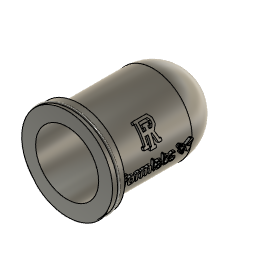
POP_body_derated (Autodesk Fusion 360 design; units mm, degrees)
Autodesk Fusion 360 part; units mm, degrees
sketch "Sketch1" plane through (0, 0, 0) normal (0, 1, 0) x (1, 0, 0)
  circle A0 centre (0, 0) radius 25.65
  circle A1 centre (0, 0) radius 31.75
  dimension "d1" = 51.3
  dimension "d2" = 6.1
  constraint coincident A0.centre A1.centre
  measures "d1" diameter of A0
extrude "Extrude1" add sketch "Sketch1" along normal blind 70 makes body 1
sketch "Sketch2" plane through (0, 0, 0) normal (0, 0, 1) x (1, 0, 0)
  line L0 (0, 0) -> (0, 97.6409) construction
  line L1 (0, 69.4626) -> (31, 69.4626)
  arc A0 (0, 95.1126) -> (-25.65, 69.4626) centre (0, 69.4626) ccw
  arc A1 (0, 101.2126) -> (-31.75, 69.4626) centre (0, 69.4626) ccw
  line L2 (0, 69.4626) -> (-31.75, 69.4626) construction
  line L3 (31, 69.4626) -> (21, 69.4626)
  line L4 (-25.65, 69.4626) -> (-31.75, 69.4626)
  line L5 (0, 95.1126) -> (0, 101.2126)
  dimension "d7" = 31.75
  dimension "d8" = 25.65
  constraint coincident L0.start origin
  constraint vertical L0
  constraint coincident L1.start L0
  constraint coincident L1.start A0.centre
  constraint perpendicular L0 L1
  constraint concentric A0 A1
  constraint coincident L1 L3.end
  constraint perpendicular L0 L2
  constraint coincident L2 A0.end
  measures "d7" radius of A1
  measures "d8" radius of A0
revolve "Revolve1" add sketch "Sketch2" angle 360 about axis through (0, 0, 0) along (0, 1, 0) bodies 1
sketch "Sketch3" plane through (0, 0, 0) normal (0, -1, 0) x (1, 0, 0)
  circle A0 centre (0, 0) radius 25.65
  circle A1 centre (0, 0) radius 31.75
  circle A2 centre (0, 0) radius 25.146 construction
  circle A3 centre (0, 0) radius 28.702 construction
  dimension "d10" = 50.292
  dimension "d11" = 57.404
  constraint coincident A0.centre A1.centre
  measures "d10" diameter of A2
  measures "d11" diameter of A3
ref_plane "WorkPlane1" through (0, 37.2468, -31.75) normal (0, 0, -1) x (1, 0, 0)
sketch "Sketch5" plane through (0, 0, 0) normal (0, -1, 0) x (1, 0, 0)
  circle A0 centre (0, 0) radius 37
  circle A1 centre (0, 0) radius 30.8058
  dimension "d31" = 74
  constraint coincident A0.centre A1.centre
  constraint concentric A0 A1
  measures "d31" diameter of A0
extrude "Extrude3" add sketch "Sketch5" against normal blind 10 bodies 1
coil "CoilPrimitive1" add diameter 74 section circle size 2 on centre turns 1.5 pitch 6.66667 right hand placed x (1, 0, 0) y (0, 0, -1) z (0, 1, 0) at (0, 0, 0) separate body makes body 2
move_body "Move1" bodies 2 to x (1, 0, 0) y (0, 1, 0) z (0, 0, 1) at (0, -1.5, 0)
combine "Combine1" operation add target body 1 tool bodies 2
sketch "Sketch7" plane through (0, 0, 0) normal (0, -1, 0) x (1, 0, 0)
  circle A0 centre (0, 0) radius 25.65
  circle A1 centre (0, 0) radius 50.9902
  spline S0 degree 3 poles (-26.163, -26.163) (-26.1604, -26.1604) (-26.1574, -26.1584) (-26.1496, -26.1548) (-26.1447, -26.1537) (-26.1307, -26.1522) (-26.1207, -26.1533) (-26.0884, -26.1593) (-26.0612, -26.1697) (-25.9436, -26.2231) (-25.8159, -26.3056) (-24.8505, -26.9737) (-23.1166, -28.4335) (-15.2241, -33.4022) (-10.4173, -34.7745) (-2.6703, -36.1642) (1.5215, -36.2078) (5.6316, -35.5568) knots 3.244354 3.244354 3.244354 3.244354 3.253489 3.253489 3.265817 3.265817 3.288767 3.288767 3.348492 3.348492 3.563904 3.563904 4.976735 4.976735 7.989432 7.989432 11.394709 11.394709 11.394709 11.394709
  spline S1 degree 3 poles (5.6316, -35.5568) (6.3802, -35.4382) (7.1261, -35.2966) (12.4413, -34.1173) (16.7708, -32.2508) (24.9958, -26.7102) (27.9306, -23.4279) (30.9522, -19.5432) (31.772, -18.3009) (32.5635, -17.1873) (32.7513, -16.9397) (32.8911, -16.8205) (32.9135, -16.8052) (32.9389, -16.796) (32.9458, -16.7943) (32.9569, -16.7943) (32.9612, -16.795) (32.9659, -16.797) (32.9666, -16.7973) (32.9672, -16.7976) knots 11.394709 11.394709 11.394709 11.394709 12.01493 12.01493 15.836449 15.836449 20.097613 20.097613 22.736598 22.736598 23.856469 23.856469 24.088678 24.088678 24.16644 24.16644 24.216158 24.216158 24.224748 24.224748 24.224748 24.224748
  arc A2 (32.9672, -16.7976) -> (-26.163, -26.163) centre (0, 0) ccw
  constraint concentric A0 A1
extrude "Extrude4" cut sketch "Sketch7" along normal blind 15 contours A1 | S0 S1 A2 bodies 1
ref_plane "WorkPlane3" through (31.75, 49.8809, 0) normal (1, 0, 0) x (0, 0, 1)
sketch "Sketch14" plane through (31.75, 0, 0) normal (1, 0, 0) x (0, 1, 0)
  spline S0 degree 3 poles (15.6914, -0.4908) (15.6818, -0.5681) (15.6432, -0.6164) (15.5562, -0.6164) knots 0 0 0 0 1 1 1 1
  spline S1 degree 3 poles (15.5562, -0.6164) (15.5369, -0.6164) (15.5079, -0.6164) (15.4596, -0.6067) knots 0 0 0 0 1 1 1 1
  spline S2 degree 3 poles (15.4596, -0.6067) (15.3244, -0.5874) (15.0637, -0.5391) (14.8125, -0.5391) knots 0 0 0 0 1 1 1 1
  spline S3 degree 3 poles (14.8125, -0.5391) (14.5614, -0.5391) (14.4069, -0.5681) (14.3006, -0.655) knots 0 0 0 0 1 1 1 1
  spline S4 degree 3 poles (14.3006, -0.655) (14.2041, -0.742) (14.1654, -0.8868) (14.1654, -1.0897) knots 0 0 0 0 1 1 1 1
  line L0 (14.1654, -1.0897) -> (14.1654, -1.6885)
  line L1 (14.1654, -1.6885) -> (15.4983, -1.6885)
  spline S5 degree 3 poles (15.4983, -1.6885) (15.5949, -1.6885) (15.6721, -1.7561) (15.6721, -1.8527) knots 0 0 0 0 1 1 1 1
  line L2 (15.6721, -1.8527) -> (15.6721, -2.8571)
  spline S6 degree 3 poles (15.6721, -2.8571) (15.6721, -2.9537) (15.5949, -3.0117) (15.4983, -3.0117) knots 0 0 0 0 1 1 1 1
  line L3 (15.4983, -3.0117) -> (14.1654, -3.0117)
  line L4 (14.1654, -3.0117) -> (14.1654, -7.213)
  spline S7 degree 3 poles (14.1654, -7.213) (14.1654, -7.3096) (14.0882, -7.3772) (13.9819, -7.3772) knots 0 0 0 0 1 1 1 1
  line L5 (13.9819, -7.3772) -> (12.4366, -7.3772)
  spline S8 degree 3 poles (12.4366, -7.3772) (12.3304, -7.3772) (12.2531, -7.3096) (12.2531, -7.213) knots 0 0 0 0 1 1 1 1
  line L6 (12.2531, -7.213) -> (12.2531, -3.0117)
  line L7 (12.2531, -3.0117) -> (11.4128, -3.0117)
  spline S9 degree 3 poles (11.4128, -3.0117) (11.3066, -3.0117) (11.2293, -2.9537) (11.2293, -2.8571) knots 0 0 0 0 1 1 1 1
  line L8 (11.2293, -2.8571) -> (11.2293, -1.8527)
  spline S10 degree 3 poles (11.2293, -1.8527) (11.2293, -1.7561) (11.3066, -1.6885) (11.4128, -1.6885) knots 0 0 0 0 1 1 1 1
  line L9 (11.4128, -1.6885) -> (12.2531, -1.6885)
  line L10 (12.2531, -1.6885) -> (12.2531, -1.0027)
  spline S11 degree 3 poles (12.2531, -1.0027) (12.2531, 0.1756) (12.8712, 0.7744) (14.1944, 0.7744) knots 0 0 0 0 1 1 1 1
  spline S12 degree 3 poles (14.1944, 0.7744) (15.054, 0.7744) (15.5466, 0.6488) (15.7108, 0.5909) knots 0 0 0 0 1 1 1 1
  spline S13 degree 3 poles (15.7108, 0.5909) (15.817, 0.5619) (15.846, 0.4653) (15.8267, 0.4074) knots 0 0 0 0 1 1 1 1
  line L11 (15.8267, 0.4074) -> (15.6914, -0.4908)
  spline S14 degree 3 poles (18.7725, -7.696) (16.2516, -7.696) (15.9329, -6.4017) (15.9329, -4.7212) knots 0 0 0 0 1 1 1 1
  spline S15 degree 3 poles (15.9329, -4.7212) (15.9329, -3.0406) (16.2516, -1.7368) (18.7725, -1.7368) knots 0 0 0 0 1 1 1 1
  spline S16 degree 3 poles (18.7725, -1.7368) (21.2933, -1.7368) (21.6217, -3.0503) (21.6217, -4.7212) knots 0 0 0 0 1 1 1 1
  spline S17 degree 3 poles (21.6217, -4.7212) (21.6217, -6.4017) (21.2933, -7.696) (18.7725, -7.696) knots 0 0 0 0 1 1 1 1
  spline S18 degree 3 poles (18.7725, -2.9827) (17.9129, -2.9827) (17.8742, -3.4849) (17.8742, -4.7212) knots 0 0 0 0 1 1 1 1
  spline S19 degree 3 poles (17.8742, -4.7212) (17.8742, -5.9575) (17.9225, -6.45) (18.7725, -6.45) knots 0 0 0 0 1 1 1 1
  spline S20 degree 3 poles (18.7725, -6.45) (19.6417, -6.45) (19.6707, -5.9478) (19.6707, -4.7212) knots 0 0 0 0 1 1 1 1
  spline S21 degree 3 poles (19.6707, -4.7212) (19.6707, -3.4753) (19.632, -2.9827) (18.7725, -2.9827) knots 0 0 0 0 1 1 1 1
  spline S22 degree 3 poles (25.6106, -3.0986) (24.9924, -3.0986) (24.4612, -3.1662) (24.3646, -3.1855) knots 0 0 0 0 1 1 1 1
  line L12 (24.3646, -3.1855) -> (24.3646, -7.3772)
  spline S23 degree 3 poles (24.3646, -7.3772) (24.3646, -7.4738) (24.297, -7.5414) (24.1908, -7.5414) knots 0 0 0 0 1 1 1 1
  line L13 (24.1908, -7.5414) -> (22.6358, -7.5414)
  spline S24 degree 3 poles (22.6358, -7.5414) (22.5392, -7.5414) (22.4619, -7.4738) (22.4619, -7.3772) knots 0 0 0 0 1 1 1 1
  line L14 (22.4619, -7.3772) -> (22.4619, -2.5867)
  spline S25 degree 3 poles (22.4619, -2.5867) (22.4619, -2.2004) (22.8096, -2.0748) (23.4567, -1.9396) knots 0 0 0 0 1 1 1 1
  spline S26 degree 3 poles (23.4567, -1.9396) (23.9783, -1.8334) (24.722, -1.7464) (25.3981, -1.7464) knots 0 0 0 0 1 1 1 1
  line L15 (25.3981, -1.7464) -> (25.5816, -1.7464)
  spline S27 degree 3 poles (25.5816, -1.7464) (25.6782, -1.7464) (25.7361, -1.7657) (25.7747, -1.814) knots 0 0 0 0 1 1 1 1
  spline S28 degree 3 poles (25.7747, -1.814) (25.8037, -1.843) (25.8327, -1.901) (25.8327, -1.9879) knots 0 0 0 0 1 1 1 1
  line L16 (25.8327, -1.9879) -> (25.8327, -2.8668)
  spline S29 degree 3 poles (25.8327, -2.8668) (25.8327, -2.9827) (25.8327, -3.0986) (25.6106, -3.0986) knots 0 0 0 0 1 1 1 1
  line L17 (35.1916, -7.5607) -> (33.6366, -7.5607)
  spline S30 degree 3 poles (33.6366, -7.5607) (33.5304, -7.5607) (33.4628, -7.4931) (33.4628, -7.3965) knots 0 0 0 0 1 1 1 1
  line L18 (33.4628, -7.3965) -> (33.4628, -3.7167)
  spline S31 degree 3 poles (33.4628, -3.7167) (33.4628, -3.1469) (33.1634, -2.9634) (32.7384, -2.9634) knots 0 0 0 0 1 1 1 1
  spline S32 degree 3 poles (32.7384, -2.9634) (32.3907, -2.9634) (31.9754, -3.0406) (31.8691, -3.06) knots 0 0 0 0 1 1 1 1
  line L19 (31.8691, -3.06) -> (31.8691, -7.3965)
  spline S33 degree 3 poles (31.8691, -7.3965) (31.8691, -7.4931) (31.7919, -7.5607) (31.6856, -7.5607) knots 0 0 0 0 1 1 1 1
  line L20 (31.6856, -7.5607) -> (30.1306, -7.5607)
  spline S34 degree 3 poles (30.1306, -7.5607) (30.0244, -7.5607) (29.9568, -7.4931) (29.9568, -7.3965) knots 0 0 0 0 1 1 1 1
  line L21 (29.9568, -7.3965) -> (29.9568, -3.7167)
  spline S35 degree 3 poles (29.9568, -3.7167) (29.9568, -3.1469) (29.7057, -2.9634) (29.2807, -2.9634) knots 0 0 0 0 1 1 1 1
  spline S36 degree 3 poles (29.2807, -2.9634) (28.9427, -2.9634) (28.4694, -3.0406) (28.3632, -3.06) knots 0 0 0 0 1 1 1 1
  line L22 (28.3632, -3.06) -> (28.3632, -7.3965)
  spline S37 degree 3 poles (28.3632, -7.3965) (28.3632, -7.4931) (28.2956, -7.5607) (28.1893, -7.5607) knots 0 0 0 0 1 1 1 1
  line L23 (28.1893, -7.5607) -> (26.6343, -7.5607)
  spline S38 degree 3 poles (26.6343, -7.5607) (26.5281, -7.5607) (26.4605, -7.4931) (26.4605, -7.3965) knots 0 0 0 0 1 1 1 1
  line L24 (26.4605, -7.3965) -> (26.4605, -2.6157)
  spline S39 degree 3 poles (26.4605, -2.6157) (26.4605, -2.2197) (26.7985, -2.0941) (27.4649, -1.9589) knots 0 0 0 0 1 1 1 1
  spline S40 degree 3 poles (27.4649, -1.9589) (28.0058, -1.8527) (28.8364, -1.7464) (29.5222, -1.7464) knots 0 0 0 0 1 1 1 1
  spline S41 degree 3 poles (29.5222, -1.7464) (30.2176, -1.7464) (30.6812, -1.9106) (30.9902, -2.1038) knots 0 0 0 0 1 1 1 1
  spline S42 degree 3 poles (30.9902, -2.1038) (31.2027, -2.0265) (32.1299, -1.7464) (33.0668, -1.7464) knots 0 0 0 0 1 1 1 1
  spline S43 degree 3 poles (33.0668, -1.7464) (34.4672, -1.7464) (35.3848, -2.0458) (35.3848, -3.456) knots 0 0 0 0 1 1 1 1
  line L25 (35.3848, -3.456) -> (35.3848, -7.4062)
  spline S44 degree 3 poles (35.3848, -7.4062) (35.3655, -7.4931) (35.2979, -7.5607) (35.1916, -7.5607) knots 0 0 0 0 1 1 1 1
  spline S45 degree 3 poles (38.5431, -7.242) (38.5431, -7.3193) (38.4948, -7.3289) (38.4561, -7.3483) knots 0 0 0 0 1 1 1 1
  spline S46 degree 3 poles (38.4561, -7.3483) (38.3402, -7.4062) (38.0698, -7.4738) (37.6738, -7.4738) knots 0 0 0 0 1 1 1 1
  spline S47 degree 3 poles (37.6738, -7.4738) (37.017, -7.4738) (36.5728, -7.1647) (36.5728, -6.3631) knots 0 0 0 0 1 1 1 1
  line L26 (36.5728, -6.3631) -> (36.5728, 0.4557)
  spline S48 degree 3 poles (36.5728, 0.4557) (36.5728, 0.5426) (36.6307, 0.6005) (36.708, 0.6199) knots 0 0 0 0 1 1 1 1
  line L27 (36.708, 0.6199) -> (37.2971, 0.7744)
  spline S49 degree 3 poles (37.2971, 0.7744) (37.3744, 0.7937) (37.442, 0.7358) (37.442, 0.6488) knots 0 0 0 0 1 1 1 1
  line L28 (37.442, 0.6488) -> (37.442, -6.3341)
  spline S50 degree 3 poles (37.442, -6.3341) (37.442, -6.7205) (37.7124, -6.7784) (37.9346, -6.7784) knots 0 0 0 0 1 1 1 1
  spline S51 degree 3 poles (37.9346, -6.7784) (38.0891, -6.7784) (38.2436, -6.7591) (38.3209, -6.7398) knots 0 0 0 0 1 1 1 1
  line L29 (38.3209, -6.7398) -> (38.3692, -6.7301)
  spline S52 degree 3 poles (38.3692, -6.7301) (38.3982, -6.7301) (38.4465, -6.7398) (38.4561, -6.8074) knots 0 0 0 0 1 1 1 1
  line L30 (38.4561, -6.8074) -> (38.5334, -7.1744)
  spline S53 degree 3 poles (38.5334, -7.1744) (38.5431, -7.2227) (38.5431, -7.2324) (38.5431, -7.242) knots 0 0 0 0 1 1 1 1
  spline S54 degree 3 poles (42.6961, -7.5318) (42.3774, -7.609) (41.8559, -7.696) (41.2667, -7.696) knots 0 0 0 0 1 1 1 1
  spline S55 degree 3 poles (41.2667, -7.696) (40.3202, -7.696) (38.7555, -7.667) (38.7555, -5.9092) knots 0 0 0 0 1 1 1 1
  spline S56 degree 3 poles (38.7555, -5.9092) (38.7555, -4.4797) (39.5379, -4.3832) (40.6486, -4.2093) knots 0 0 0 0 1 1 1 1
  line L31 (40.6486, -4.2093) -> (42.7251, -3.8713)
  line L32 (42.7251, -3.8713) -> (42.7251, -3.3594)
  spline S57 degree 3 poles (42.7251, -3.3594) (42.7251, -3.0117) (42.7155, -2.7316) (42.3291, -2.5867) knots 0 0 0 0 1 1 1 1
  spline S58 degree 3 poles (42.3291, -2.5867) (42.1166, -2.4998) (41.8172, -2.4611) (41.3343, -2.4611) knots 0 0 0 0 1 1 1 1
  spline S59 degree 3 poles (41.3343, -2.4611) (40.494, -2.4611) (39.7697, -2.664) (39.3061, -2.7702) knots 0 0 0 0 1 1 1 1
  spline S60 degree 3 poles (39.3061, -2.7702) (39.1998, -2.7895) (39.1515, -2.7799) (39.1322, -2.693) knots 0 0 0 0 1 1 1 1
  line L33 (39.1322, -2.693) -> (39.0356, -2.21)
  spline S61 degree 3 poles (39.0356, -2.21) (39.0163, -2.1135) (39.1129, -2.0652) (39.1419, -2.0555) knots 0 0 0 0 1 1 1 1
  spline S62 degree 3 poles (39.1419, -2.0555) (39.4896, -1.9299) (40.4361, -1.7175) (41.4309, -1.7175) knots 0 0 0 0 1 1 1 1
  spline S63 degree 3 poles (41.4309, -1.7175) (42.2132, -1.7175) (42.7155, -1.8237) (43.0342, -1.9975) knots 0 0 0 0 1 1 1 1
  spline S64 degree 3 poles (43.0342, -1.9975) (43.5944, -2.2873) (43.604, -2.7992) (43.604, -3.3111) knots 0 0 0 0 1 1 1 1
  line L34 (43.604, -3.3111) -> (43.604, -6.4114)
  spline S65 degree 3 poles (43.604, -6.4114) (43.604, -7.1841) (43.4495, -7.3579) (42.6961, -7.5318) knots 0 0 0 0 1 1 1 1
  line L35 (42.7348, -4.557) -> (40.6003, -4.9144)
  spline S66 degree 3 poles (40.6003, -4.9144) (40.1174, -5.0013) (39.6538, -5.0786) (39.6538, -5.8705) knots 0 0 0 0 1 1 1 1
  spline S67 degree 3 poles (39.6538, -5.8705) (39.6538, -6.9523) (40.552, -7.0295) (41.2764, -7.0295) knots 0 0 0 0 1 1 1 1
  spline S68 degree 3 poles (41.2764, -7.0295) (41.7593, -7.0295) (42.2712, -6.9619) (42.7348, -6.8171) knots 0 0 0 0 1 1 1 1
  line L36 (42.7348, -6.8171) -> (42.7348, -4.557)
  spline S69 degree 3 poles (45.7288, -1.8527) (46.0283, -1.7657) (46.8878, -1.5533) (47.5833, -1.5533) knots 0 0 0 0 1 1 1 1
  spline S70 degree 3 poles (47.5833, -1.5533) (49.399, -1.5533) (49.9109, -2.4708) (49.9109, -4.5184) knots 0 0 0 0 1 1 1 1
  spline S71 degree 3 poles (49.9109, -4.5184) (49.9109, -6.6239) (49.3314, -7.5125) (47.3418, -7.5125) knots 0 0 0 0 1 1 1 1
  spline S72 degree 3 poles (47.3418, -7.5125) (46.5595, -7.5125) (45.8544, -7.3869) (45.4874, -7.2613) knots 0 0 0 0 1 1 1 1
  spline S73 degree 3 poles (45.4874, -7.2613) (44.9369, -7.0778) (44.9176, -6.8074) (44.9176, -6.4114) knots 0 0 0 0 1 1 1 1
  line L37 (44.9176, -6.4114) -> (44.9176, 0.4653)
  spline S74 degree 3 poles (44.9176, 0.4653) (44.9176, 0.5523) (44.9658, 0.5812) (45.0528, 0.6102) knots 0 0 0 0 1 1 1 1
  line L38 (45.0528, 0.6102) -> (45.6419, 0.7647)
  spline S75 degree 3 poles (45.6419, 0.7647) (45.7385, 0.7937) (45.7868, 0.6971) (45.7868, 0.6392) knots 0 0 0 0 1 1 1 1
  line L39 (45.7868, 0.6392) -> (45.7868, -1.2539)
  line L40 (45.7868, -1.2539) -> (45.7288, -1.8527)
  spline S76 degree 3 poles (47.4384, -2.2583) (46.8396, -2.2583) (45.98, -2.4611) (45.7868, -2.5191) knots 0 0 0 0 1 1 1 1
  line L41 (45.7868, -2.5191) -> (45.7868, -6.6432)
  spline S77 degree 3 poles (45.7868, -6.6432) (45.9027, -6.6818) (46.4919, -6.8364) (47.3225, -6.8364) knots 0 0 0 0 1 1 1 1
  spline S78 degree 3 poles (47.3225, -6.8364) (48.5877, -6.8364) (49.0127, -6.2569) (49.0127, -4.5473) knots 0 0 0 0 1 1 1 1
  spline S79 degree 3 poles (49.0127, -4.5473) (49.0127, -2.7992) (48.7036, -2.2583) (47.4384, -2.2583) knots 0 0 0 0 1 1 1 1
  spline S80 degree 3 poles (52.3834, -7.696) (51.4176, -7.696) (50.587, -7.4062) (50.4421, -7.3483) knots 0 0 0 0 1 1 1 1
  spline S81 degree 3 poles (50.4421, -7.3483) (50.3842, -7.3289) (50.3359, -7.2903) (50.3648, -7.1744) knots 0 0 0 0 1 1 1 1
  line L42 (50.3648, -7.1744) -> (50.4614, -6.7591)
  spline S82 degree 3 poles (50.4614, -6.7591) (50.4807, -6.6818) (50.5194, -6.6142) (50.6353, -6.6625) knots 0 0 0 0 1 1 1 1
  spline S83 degree 3 poles (50.6353, -6.6625) (50.6643, -6.6722) (51.4659, -6.9716) (52.4028, -6.9716) knots 0 0 0 0 1 1 1 1
  spline S84 degree 3 poles (52.4028, -6.9716) (53.33, -6.9716) (53.8708, -6.6818) (53.8708, -6.0154) knots 0 0 0 0 1 1 1 1
  spline S85 degree 3 poles (53.8708, -6.0154) (53.8708, -5.1172) (53.1658, -5.1462) (52.3158, -5.0206) knots 0 0 0 0 1 1 1 1
  spline S86 degree 3 poles (52.3158, -5.0206) (51.775, -4.9337) (50.4035, -4.8371) (50.4035, -3.4077) knots 0 0 0 0 1 1 1 1
  spline S87 degree 3 poles (50.4035, -3.4077) (50.4035, -2.0072) (51.6687, -1.7175) (52.6249, -1.7175) knots 0 0 0 0 1 1 1 1
  spline S88 degree 3 poles (52.6249, -1.7175) (53.5714, -1.7175) (54.3054, -1.9106) (54.4213, -1.9493) knots 0 0 0 0 1 1 1 1
  spline S89 degree 3 poles (54.4213, -1.9493) (54.4986, -1.9686) (54.5276, -2.0169) (54.5179, -2.0748) knots 0 0 0 0 1 1 1 1
  line L43 (54.5179, -2.0748) -> (54.4407, -2.5577)
  spline S90 degree 3 poles (54.4407, -2.5577) (54.431, -2.6253) (54.3924, -2.6447) (54.3248, -2.6447) knots 0 0 0 0 1 1 1 1
  spline S91 degree 3 poles (54.3248, -2.6447) (54.1702, -2.6253) (53.3589, -2.4418) (52.7118, -2.4418) knots 0 0 0 0 1 1 1 1
  spline S92 degree 3 poles (52.7118, -2.4418) (51.9198, -2.4418) (51.2631, -2.6543) (51.2631, -3.3401) knots 0 0 0 0 1 1 1 1
  spline S93 degree 3 poles (51.2631, -3.3401) (51.2631, -4.0741) (52.0068, -4.161) (52.6925, -4.2479) knots 0 0 0 0 1 1 1 1
  spline S94 degree 3 poles (52.6925, -4.2479) (53.6777, -4.3735) (54.7401, -4.4508) (54.7401, -5.9285) knots 0 0 0 0 1 1 1 1
  spline S95 degree 3 poles (54.7401, -5.9285) (54.7497, -7.3483) (53.6487, -7.696) (52.3834, -7.696) knots 0 0 0 0 1 1 1 1
  spline S96 degree 3 poles (69.1696, -0.5391) (69.0441, -0.9544) (68.7543, -1.2828) (68.5225, -1.6402) knots 0 0 0 0 1 1 1 1
  spline S97 degree 3 poles (68.5225, -1.6402) (67.943, -2.5191) (67.3538, -3.398) (66.7743, -4.2769) knots 0 0 0 0 1 1 1 1
  spline S98 degree 3 poles (66.7743, -4.2769) (66.7647, -4.2962) (66.755, -4.3155) (66.7357, -4.3445) knots 0 0 0 0 1 1 1 1
  spline S99 degree 3 poles (66.7357, -4.3445) (66.9289, -4.4797) (67.122, -4.5956) (67.3056, -4.7405) knots 0 0 0 0 1 1 1 1
  spline S100 degree 3 poles (67.3056, -4.7405) (67.3828, -4.7985) (67.4601, -4.8757) (67.5084, -4.953) knots 0 0 0 0 1 1 1 1
  spline S101 degree 3 poles (67.5084, -4.953) (67.6243, -5.1655) (67.5567, -5.4069) (67.3635, -5.5615) knots 0 0 0 0 1 1 1 1
  spline S102 degree 3 poles (67.3635, -5.5615) (66.6971, -6.112) (66.021, -6.6432) (65.3642, -7.2034) knots 0 0 0 0 1 1 1 1
  spline S103 degree 3 poles (65.3642, -7.2034) (65.0165, -7.5028) (64.6012, -7.3289) (64.4757, -6.9716) knots 0 0 0 0 1 1 1 1
  spline S104 degree 3 poles (64.4757, -6.9716) (64.0024, -5.5808) (63.5195, -4.19) (63.0366, -2.7992) knots 0 0 0 0 1 1 1 1
  spline S105 degree 3 poles (63.0366, -2.7992) (63.0269, -2.7799) (63.0173, -2.7509) (62.9979, -2.7026) knots 0 0 0 0 1 1 1 1
  spline S106 degree 3 poles (62.9979, -2.7026) (62.9593, -2.7992) (62.9303, -2.8861) (62.9014, -2.9634) knots 0 0 0 0 1 1 1 1
  spline S107 degree 3 poles (62.9014, -2.9634) (62.4474, -4.2769) (61.9935, -5.5904) (61.5492, -6.904) knots 0 0 0 0 1 1 1 1
  spline S108 degree 3 poles (61.5492, -6.904) (61.5299, -6.9523) (61.5202, -7.0006) (61.5009, -7.0392) knots 0 0 0 0 1 1 1 1
  spline S109 degree 3 poles (61.5009, -7.0392) (61.3753, -7.3676) (60.9793, -7.4835) (60.7089, -7.2613) knots 0 0 0 0 1 1 1 1
  spline S110 degree 3 poles (60.7089, -7.2613) (60.4385, -7.0392) (60.168, -6.817) (59.888, -6.5949) knots 0 0 0 0 1 1 1 1
  spline S111 degree 3 poles (59.888, -6.5949) (59.4823, -6.2665) (59.0863, -5.9285) (58.6807, -5.6098) knots 0 0 0 0 1 1 1 1
  spline S112 degree 3 poles (58.6807, -5.6098) (58.3523, -5.349) (58.3619, -4.982) (58.7193, -4.7405) knots 0 0 0 0 1 1 1 1
  spline S113 degree 3 poles (58.7193, -4.7405) (58.9221, -4.6053) (59.1153, -4.4701) (59.3278, -4.3349) knots 0 0 0 0 1 1 1 1
  spline S114 degree 3 poles (59.3278, -4.3349) (59.2505, -4.219) (59.1732, -4.1127) (59.1056, -3.9968) knots 0 0 0 0 1 1 1 1
  spline S115 degree 3 poles (59.1056, -3.9968) (58.4102, -2.9827) (57.7148, -1.9589) (57.0194, -0.9448) knots 0 0 0 0 1 1 1 1
  spline S116 degree 3 poles (57.0194, -0.9448) (56.7683, -0.5778) (56.8552, 0.021) (57.2995, 0.2335) knots 0 0 0 0 1 1 1 1
  spline S117 degree 3 poles (57.2995, 0.2335) (57.541, 0.3591) (57.7728, 0.504) (58.0046, 0.6295) knots 0 0 0 0 1 1 1 1
  spline S118 degree 3 poles (58.0046, 0.6295) (58.275, 0.7744) (58.5551, 0.7744) (58.8255, 0.6199) knots 0 0 0 0 1 1 1 1
  spline S119 degree 3 poles (58.8255, 0.6199) (60.1874, -0.1818) (61.5395, -0.9834) (62.9014, -1.7947) knots 0 0 0 0 1 1 1 1
  spline S120 degree 3 poles (62.9014, -1.7947) (62.9786, -1.843) (63.0366, -1.843) (63.1235, -1.7947) knots 0 0 0 0 1 1 1 1
  spline S121 degree 3 poles (63.1235, -1.7947) (64.4757, -0.9834) (65.8182, -0.1818) (67.1703, 0.6199) knots 0 0 0 0 1 1 1 1
  spline S122 degree 3 poles (67.1703, 0.6199) (67.4601, 0.7937) (67.7498, 0.7937) (68.0396, 0.6295) knots 0 0 0 0 1 1 1 1
  spline S123 degree 3 poles (68.0396, 0.6295) (68.2617, 0.504) (68.4839, 0.3687) (68.7157, 0.2529) knots 0 0 0 0 1 1 1 1
  spline S124 degree 3 poles (68.7157, 0.2529) (68.9571, 0.1273) (69.0634, -0.0755) (69.1503, -0.3073) knots 0 0 0 0 1 1 1 1
  spline S125 degree 3 poles (69.1503, -0.3073) (69.1599, -0.3266) (69.1599, -0.3556) (69.1696, -0.3846) knots 0 0 0 0 1 1 1 1
  spline S126 degree 3 poles (69.1696, -0.3846) (69.1696, -0.4232) (69.1696, -0.4812) (69.1696, -0.5391) knots 0 0 0 0 1 1 1 1
  spline S127 degree 3 poles (68.4163, -0.8675) (68.4163, -0.8579) (68.4066, -0.8579) (68.4066, -0.8482) knots 0 0 0 0 1 1 1 1
  spline S128 degree 3 poles (68.4066, -0.8482) (66.813, -1.3118) (65.2194, -1.7754) (63.6064, -2.239) knots 0 0 0 0 1 1 1 1
  spline S129 degree 3 poles (63.6064, -2.239) (64.524, -2.8475) (65.4125, -3.4463) (66.3204, -4.0451) knots 0 0 0 0 1 1 1 1
  spline S130 degree 3 poles (66.3204, -4.0451) (67.0255, -2.9827) (67.7209, -1.9299) (68.4163, -0.8675) knots 0 0 0 0 1 1 1 1
  spline S131 degree 3 poles (62.4378, -2.239) (60.8345, -1.7754) (59.2602, -1.3118) (57.6859, -0.8579) knots 0 0 0 0 1 1 1 1
  spline S132 degree 3 poles (57.6859, -0.8579) (57.6859, -0.8675) (57.6762, -0.8675) (57.6762, -0.8772) knots 0 0 0 0 1 1 1 1
  spline S133 degree 3 poles (57.6762, -0.8772) (58.3909, -1.9203) (59.096, -2.9634) (59.8203, -4.0065) knots 0 0 0 0 1 1 1 1
  spline S134 degree 3 poles (59.8203, -4.0065) (60.6896, -3.4173) (61.5589, -2.8378) (62.4378, -2.239) knots 0 0 0 0 1 1 1 1
  spline S135 degree 3 poles (61.0566, -6.7977) (61.4043, -5.7643) (61.752, -4.7502) (62.0997, -3.736) knots 0 0 0 0 1 1 1 1
  spline S136 degree 3 poles (62.0997, -3.736) (62.0611, -3.7457) (62.0418, -3.7747) (62.0321, -3.794) knots 0 0 0 0 1 1 1 1
  spline S137 degree 3 poles (62.0321, -3.794) (61.6941, -4.2576) (61.356, -4.7212) (61.0276, -5.1848) knots 0 0 0 0 1 1 1 1
  spline S138 degree 3 poles (61.0276, -5.1848) (60.9793, -5.2524) (60.9407, -5.3103) (60.8924, -5.3683) knots 0 0 0 0 1 1 1 1
  spline S139 degree 3 poles (60.8924, -5.3683) (60.6799, -5.6291) (60.2743, -5.6194) (60.0811, -5.349) knots 0 0 0 0 1 1 1 1
  spline S140 degree 3 poles (60.0811, -5.349) (59.9459, -5.1558) (59.8203, -4.9626) (59.6755, -4.7598) knots 0 0 0 0 1 1 1 1
  spline S141 degree 3 poles (59.6755, -4.7598) (59.4726, -4.895) (59.2698, -5.0303) (59.067, -5.1655) knots 0 0 0 0 1 1 1 1
  spline S142 degree 3 poles (59.067, -5.1655) (59.7334, -5.716) (60.3902, -6.2472) (61.0566, -6.7977) knots 0 0 0 0 1 1 1 1
  spline S143 degree 3 poles (57.541, -0.2494) (58.6903, -0.5874) (59.8107, -0.9158) (60.9311, -1.2442) knots 0 0 0 0 1 1 1 1
  spline S144 degree 3 poles (60.9311, -1.2442) (60.9214, -1.2152) (60.9021, -1.1959) (60.8924, -1.1862) knots 0 0 0 0 1 1 1 1
  spline S145 degree 3 poles (60.8924, -1.1862) (60.1198, -0.7323) (59.3471, -0.2687) (58.5744, 0.1852) knots 0 0 0 0 1 1 1 1
  spline S146 degree 3 poles (58.5744, 0.1852) (58.4875, 0.2335) (58.3909, 0.2335) (58.304, 0.1852) knots 0 0 0 0 1 1 1 1
  spline S147 degree 3 poles (58.304, 0.1852) (58.1205, 0.079) (57.937, -0.0176) (57.7631, -0.1238) knots 0 0 0 0 1 1 1 1
  spline S148 degree 3 poles (57.7631, -0.1238) (57.6955, -0.1625) (57.6279, -0.2011) (57.541, -0.2494) knots 0 0 0 0 1 1 1 1
  spline S149 degree 3 poles (61.5782, -3.5042) (61.5685, -3.4946) (61.5685, -3.4946) (61.5588, -3.4849) knots 0 0 0 0 1 1 1 1
  spline S150 degree 3 poles (61.5588, -3.4849) (61.0856, -3.8036) (60.6123, -4.132) (60.1294, -4.4508) knots 0 0 0 0 1 1 1 1
  spline S151 degree 3 poles (60.1294, -4.4508) (60.255, -4.6343) (60.3805, -4.8081) (60.5061, -4.9916) knots 0 0 0 0 1 1 1 1
  spline S152 degree 3 poles (60.5061, -4.9916) (60.8635, -4.4894) (61.2208, -3.9968) (61.5782, -3.5042) knots 0 0 0 0 1 1 1 1
emboss "Emboss8" depth 2 profiles "Sketch14" section 1 onto face at (31.5922, 30, -3.1613) on bodies 1 bodies 1
sketch "URI_logo" plane through (31.75, -0.7168, -52.8588) normal (1, 0, 0) x (0, 1, 0)
  line L0 (78.7402, 18.9961) -> (7.874, 18.9961)
  line L1 (7.874, 25.689) -> (7.874, 3.937)
  line L2 (29.3701, 10.6299) -> (7.874, 10.6299)
  line L3 (18.5004, 18.9961) -> (18.5004, 3.937)
  line L4 (67.2441, 23.1791) -> (67.2441, 25.689)
  line L5 (29.3701, 3.937) -> (29.3701, 18.9961)
  line L6 (29.3701, 8.9567) -> (7.874, 8.9567)
  line L7 (39.5596, 61.9109) -> (39.5596, 69.0155)
  line L8 (46.7717, 17.3228) -> (7.874, 17.3228)
  line L9 (46.7717, 12.3031) -> (7.874, 12.3031)
  line L10 (64.1732, 3.937) -> (64.1732, 5.6102)
  line L11 (29.3701, 10.6299) -> (78.7402, 10.6299)
  line L12 (78.7402, 7.2835) -> (73.622, 7.2835)
  line L13 (25.3539, 18.9961) -> (25.3539, 3.937)
  line L14 (46.7717, 25.689) -> (46.7717, 3.937)
  line L15 (80.7087, 58.4646) -> (76.7717, 58.4646)
  line L16 (5.9055, 58.4646) -> (9.8425, 58.4646)
  line L17 (45.6563, 63.8888) -> (44.3969, 63.8888)
  line L18 (39.6063, 25.689) -> (39.6063, 10.6299)
  line L19 (43.3071, 1.9685) -> (43.3071, 5.9055)
  line L20 (7.874, 3.937) -> (7.874, 112.9921)
  line L21 (34.6481, 71.5623) -> (37.1596, 71.5623)
  line L22 (35.9596, 75.4695) -> (40.7596, 75.4695)
  line L23 (40.7596, 61.9109) -> (39.5596, 61.9109)
  line L24 (40.7596, 59.9071) -> (40.7596, 61.9109)
  line L25 (43.3071, 114.9606) -> (43.3071, 111.0236)
  line L26 (37.1596, 71.5623) -> (37.1596, 73.4695)
  line L27 (43.0019, 73.4695) -> (43.0019, 75.4695)
  line L28 (31.239, 61.9109) -> (35.611, 61.9109)
  line L29 (46.7717, 13.9764) -> (7.874, 13.9764)
  line L30 (43.3071, 112.9921) -> (43.3071, 114.9606)
  line L31 (7.874, 25.689) -> (78.7402, 25.689)
  line L32 (7.874, 5.6102) -> (78.7402, 5.6102)
  line L33 (29.3701, 7.2835) -> (7.874, 7.2835)
  line L34 (35.611, 61.9109) -> (35.611, 63.8888)
  line L35 (41.7007, 77.5514) -> (34.6481, 77.5514)
  line L36 (78.7402, 78.1496) -> (80.7087, 78.1496)
  line L37 (45.0057, 72.3535) -> (45.0057, 76.2502)
  line L38 (78.7402, 3.937) -> (7.874, 3.937)
  line L39 (35.611, 63.8888) -> (34.5961, 63.8888)
  line L40 (33.4646, 12.3031) -> (33.4646, 18.9961)
  line L41 (80.7087, 114.9606) -> (80.7087, 1.9685)
  line L42 (21.1811, 18.9961) -> (21.1811, 25.689)
  line L43 (10.9449, 18.9961) -> (10.9449, 3.937)
  line L44 (78.7402, 23.1791) -> (46.7717, 23.1791)
  line L45 (45.6563, 61.9109) -> (45.6563, 63.8888)
  line L46 (46.7717, 15.6496) -> (7.874, 15.6496)
  line L47 (34.6481, 77.5514) -> (34.6481, 71.5623)
  line L48 (35.9596, 59.9071) -> (40.7596, 59.9071)
  line L49 (73.622, 5.6102) -> (73.622, 10.6299)
  line L50 (42.2741, 69.1707) -> (45.0057, 72.3535)
  line L51 (43.0019, 61.9109) -> (45.6563, 61.9109)
  line L52 (80.7087, 1.9685) -> (5.9055, 1.9685)
  line L53 (34.5961, 69.0155) -> (37.1596, 69.0155)
  line L54 (39.5596, 69.0155) -> (40.1465, 69.0155)
  line L55 (35.9596, 73.4695) -> (35.9596, 75.4695)
  line L56 (7.874, 38.7795) -> (5.9055, 38.7795)
  line L57 (23.622, 112.9921) -> (23.622, 114.9606)
  line L58 (39.5596, 71.5623) -> (41.7007, 71.5623)
  line L59 (32.6443, 77.5774) -> (32.6443, 63.8888)
  line L60 (45.0057, 76.2502) -> (42.7937, 79.4772)
  line L61 (40.7596, 73.4695) -> (39.5596, 73.4695)
  line L62 (43.3071, 3.937) -> (43.3071, 1.9685)
  line L63 (7.874, 58.4646) -> (5.9055, 58.4646)
  line L64 (39.5596, 73.4695) -> (39.5596, 71.5623)
  line L65 (78.7402, 19.0945) -> (80.7087, 19.0945)
  line L66 (23.622, 3.937) -> (23.622, 1.9685)
  line L67 (43.0019, 75.4695) -> (41.7007, 77.5514)
  line L68 (5.9055, 1.9685) -> (5.9055, 114.9606)
  line L69 (35.9596, 61.9109) -> (35.9596, 59.9071)
  line L70 (31.239, 63.8888) -> (31.239, 61.9109)
  line L71 (7.874, 78.1496) -> (5.9055, 78.1496)
  line L72 (78.7402, 58.4646) -> (80.7087, 58.4646)
  line L73 (31.265, 77.5774) -> (32.6443, 77.5774)
  line L74 (37.1596, 61.9109) -> (35.9596, 61.9109)
  line L75 (37.1596, 73.4695) -> (35.9596, 73.4695)
  line L76 (62.9921, 3.937) -> (62.9921, 1.9685)
  line L77 (34.5961, 63.8888) -> (34.5961, 69.0155)
  line L78 (78.7402, 38.7795) -> (80.7087, 38.7795)
  line L79 (7.874, 112.9921) -> (78.7402, 112.9921)
  line L80 (78.7402, 97.8346) -> (80.7087, 97.8346)
  line L81 (41.7007, 71.5623) -> (43.0019, 73.4695)
  line L82 (37.1596, 69.0155) -> (37.1596, 61.9109)
  line L83 (78.7402, 112.9921) -> (78.7402, 3.937)
  line L84 (44.3969, 63.8888) -> (42.2741, 69.1707)
  line L85 (40.7596, 75.4695) -> (40.7596, 73.4695)
  line L86 (62.9921, 112.9921) -> (62.9921, 114.9606)
  line L87 (5.9055, 114.9606) -> (80.7087, 114.9606)
  line L88 (42.7937, 79.4772) -> (31.265, 79.4772)
  line L89 (7.874, 97.8346) -> (5.9055, 97.8346)
  line L90 (32.6443, 63.8888) -> (31.239, 63.8888)
  line L91 (7.874, 19.0945) -> (5.9055, 19.0945)
  line L92 (31.265, 79.4772) -> (31.265, 77.5774)
  line L93 (40.1465, 69.0155) -> (43.0019, 61.9109)
emboss "Emboss9" depth 2 profiles "URI_logo" section 1 contours L7 L17 L23 L24 L28 L34 L37 L39 L45 L48 L50 L51 L53 L54 L59 L60 L69 L70 L73 L74 L77 L82 L84 L88 L90 L92 L93 onto face at (31.7444, 62.9682, -0.5982) on bodies 1 bodies 1
